# Autodesk Inventor part: Shaft
Saved by Autodesk Inventor 2015 (Build 190159000, 159)
## iProperties
Created: 2013-07-10
Part Number: Shaft
Material: Steel
Document SubType Name: Modeling
Designer: Michael Green
Density: 1 g/cm^3
Appearance: Steel
CustomPartVersion: 1
Author: Michael Green
Autodesk Inventor part; units mm, degrees
ref_plane "Start Plane" through (0, 0, 0) normal (1, 0, 0) x (0, 1, 0)
ref_plane "XZ Plane" through (0, 0, 0) normal (0, 1, 0) x (-1, 0, 0)
ref_plane "XY Plane" through (0, 0, 0) normal (0, 0, 1) x (1, 0, 0)
sketch "Main Sketch" plane through (0, 0, 0) normal (0, 0, 1) x (1, 0, 0)
  line L0 (0, 0) -> (80, 0)
  line L1 (0, 0) -> (0, 3)
  line L2 (80, 3) -> (80, 0)
  line L3 (0, 3) -> (80, 3)
  dimension "d3" = 6
  constraints: 8 end point, 3 horizontal, 2 vertical
  measures "d3" diameter of L3 L0
revolve "Revolution1" add sketch "Main Sketch" angle 360 about axis through (0, 0, 0) along (1, 0, 0)
chamfer "Chamfer1" distance 0.5 angle 45 1 edges at (0, -3, 0) measured on face at (53.3333, 2.9612, -0.4812)
chamfer "Chamfer2" distance 0.5 angle 45 1 edges at (80, -3, 0) measured on face at (53.5, 2.9903, -0.2414)
body "Solid1"
